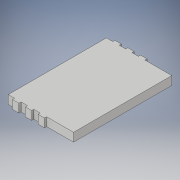
# Autodesk Inventor part: ramp
Saved by Autodesk Inventor 2019 (Build 230136000, 136)
## iProperties
Created: 2019-11-04
Part Number: ramp
Material: Generic
Document SubType Name: Modeling
Designer: shrey
Density: 1 g/cm^3
Appearance: Default
Author: shrey
Autodesk Inventor part; units mm, degrees
ref_plane "YZ Plane" through (0, 0, 0) normal (1, 0, 0) x (0, 1, 0)
ref_plane "XZ Plane" through (0, 0, 0) normal (0, 1, 0) x (-1, 0, 0)
ref_plane "XY Plane" through (0, 0, 0) normal (0, 0, 1) x (1, 0, 0)
sketch "Sketch1" plane through (0, 0, 0) normal (0, 1, 0) x (-1, 0, 0)
  line L0 (97.155, 146.05) -> (-97.155, 146.05)
  line L1 (-97.155, 146.05) -> (-97.155, -146.05)
  line L2 (-97.155, -146.05) -> (97.155, -146.05)
  line L3 (97.155, -146.05) -> (97.155, 146.05)
  line L4 (97.155, 146.05) -> (-97.155, -146.05) construction
  line L5 (-97.155, 146.05) -> (97.155, -146.05) construction
  line L6 (97.155, -146.05) -> (78.105, -146.05)
  line L7 (78.105, -146.05) -> (59.055, -146.05)
  line L8 (59.055, -146.05) -> (59.055, -152.4)
  line L9 (59.055, -152.4) -> (78.105, -152.4)
  line L10 (78.105, -152.4) -> (78.105, -146.05)
  line L11 (40.005, -146.05) -> (20.955, -146.05)
  line L12 (40.005, -152.4) -> (40.005, -146.05)
  line L13 (20.955, -146.05) -> (20.955, -152.4)
  line L14 (20.955, -152.4) -> (40.005, -152.4)
  line L15 (1.905, -146.05) -> (-17.145, -146.05)
  line L16 (1.905, -152.4) -> (1.905, -146.05)
  line L17 (-17.145, -146.05) -> (-17.145, -152.4)
  line L18 (-17.145, -152.4) -> (1.905, -152.4)
  line L19 (78.105, 146.05) -> (59.055, 146.05)
  line L20 (59.055, 146.05) -> (59.055, 152.4)
  line L21 (59.055, 152.4) -> (78.105, 152.4)
  line L22 (78.105, 152.4) -> (78.105, 146.05)
  line L23 (40.005, 146.05) -> (20.955, 146.05)
  line L24 (40.005, 152.4) -> (40.005, 146.05)
  line L25 (20.955, 146.05) -> (20.955, 152.4)
  line L26 (20.955, 152.4) -> (40.005, 152.4)
  line L27 (1.905, 146.05) -> (-17.145, 146.05)
  line L28 (1.905, 152.4) -> (1.905, 146.05)
  line L29 (-17.145, 146.05) -> (-17.145, 152.4)
  line L30 (-17.145, 152.4) -> (1.905, 152.4)
  point P0 (0, 0)
  dimension "d0" = 292.1
  dimension "d1" = 194.31
  dimension "d2" = 19.05
  dimension "d3" = 19.05
  dimension "d4" = 6.35
  dimension "d7" = 38.1
  constraints: 62 end point, 4 parallel, 3 horizontal, 2 midpoint, 2 perpendicular, 1 point on line, 16 other
  measures "d0" distance of L0.end L1.end
  measures "d1" distance of L0.start L0.end
  measures "d2" distance of L2.end L6.end
  measures "d3" distance of L9.end L8.end
  measures "d4" distance of L7.end L8.end
  measures "d7" distance of L6.end L11.start
extrude "Extrusion1" add sketch "Sketch1" along normal blind 25.4
body "Solid1"
